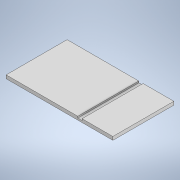
# Autodesk Inventor part: test
Saved by Autodesk Inventor 2021.1 (Build 251245010, 245A)
## iProperties
Created: 2021-07-25
Part Number: test
Material: Типовые
Document SubType Name: Modeling
Designer: User
Density: 1 g/cm^3
Appearance: По умолчанию
Author: User
Autodesk Inventor part; units mm, degrees
ref_plane "YZ Plane" through (0, 0, 0) normal (1, 0, 0) x (0, 1, 0)
ref_plane "XZ Plane" through (0, 0, 0) normal (0, 1, 0) x (-1, 0, 0)
ref_plane "XY Plane" through (0, 0, 0) normal (0, 0, 1) x (1, 0, 0)
sketch "Эскиз1" plane through (0, 0, 0) normal (0, 1, 0) x (-1, 0, 0)
  line L0 (-35, -20) -> (35, -20)
  line L1 (35, -20) -> (35, 20)
  line L2 (35, 20) -> (-35, 20)
  line L3 (-35, 20) -> (-35, -20)
  line L4 (-35, -20) -> (35, 20) construction
  line L5 (35, -20) -> (-35, 20) construction
  point P0 (0, 0)
  dimension "d0" = 70
  dimension "d1" = 40
  constraints: 12 end point, 2 midpoint, 2 parallel, 1 horizontal, 1 perpendicular
  measures "d0" distance of L2.end L1.end
  measures "d1" distance of L1.end L0.end
extrude "Выдавливание1" add sketch "Эскиз1" along normal blind 2.2
sketch "Эскиз2" plane through (0, 2.2, 0) normal (0, 1, 0) x (1, 0, 0)
  line L0 (-35, -20) -> (35, -20) projected
  line L1 (35, 20) -> (-35, 20) projected
  line L2 (12.0013, -20) -> (14.8088, -20)
  line L3 (14.8088, -20) -> (14.8088, 20)
  line L4 (14.8088, 20) -> (12.0013, 20)
  line L5 (12.0013, 20) -> (12.0013, -20)
  point P0 (0, 0)
  constraints: 8 end point, 2 parallel, 2 point on line, 1 horizontal, 1 perpendicular
extrude "Выдавливание2" cut sketch "Эскиз2" against normal blind 1
